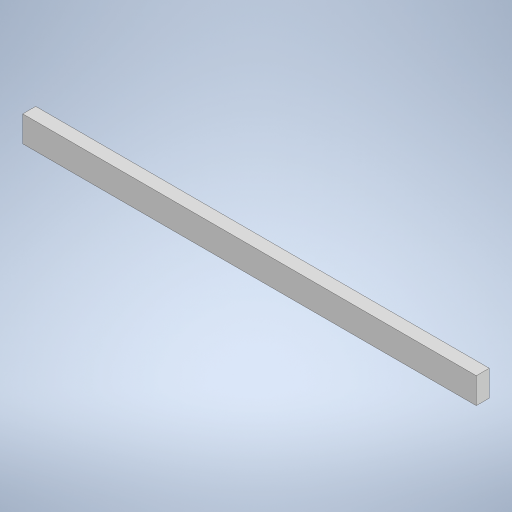
# Autodesk Inventor part: tail vertical rod
Saved by Autodesk Inventor 2024 (Build 280153000, 153)
## iProperties
Created: 2023-07-07
Part Number: tail vertical rod
Material: Generic
Document SubType Name: Modeling
Designer: USER
Density: 1 g/cm^3
Appearance: Default
Author: USER
Autodesk Inventor part; units mm, degrees
ref_plane "YZ Plane" through (0, 0, 0) normal (1, 0, 0) x (0, 1, 0)
ref_plane "XZ Plane" through (0, 0, 0) normal (0, 1, 0) x (-1, 0, 0)
ref_plane "XY Plane" through (0, 0, 0) normal (0, 0, 1) x (1, 0, 0)
sketch "Sketch1" plane through (0, 0, 0) normal (0, 0, 1) x (1, 0, 0)
  line L0 (150, 5) -> (-150, 5)
  line L1 (-150, 5) -> (-150, -5)
  line L2 (-150, -5) -> (150, -5)
  line L3 (150, -5) -> (150, 5)
  point P0 (0, 0)
  constraints: 8 end point, 2 parallel, 1 horizontal, 1 perpendicular
extrude "Extrusion1" add sketch "Sketch1" along normal blind 5
sketch "Sketch2" plane through (150, -5, 0) normal (1, 0, 0) x (0, 0, -1)
  line L0 (0, 0) -> (0, 10) projected
  line L1 (0, 10) -> (-5, 10) projected
  line L2 (-5, 0) -> (-5, 10) projected
  line L3 (0, 0) -> (-5, 0) projected
  point P0 (0, 5)
extrude "Extrusion2" cut sketch "Sketch2" against normal blind 150
sketch "Sketch3" plane through (0, -5, 0) normal (1, 0, 0) x (0, 0, -1)
  line L0 (0, 10) -> (0, 0) projected
  line L1 (-5, 10) -> (0, 10) projected
  line L2 (-5, 0) -> (-5, 10) projected
  line L3 (0, 0) -> (-5, 0) projected
  point P0 (0, 5)
extrude "Extrusion3" add sketch "Sketch3" along normal blind 50
sketch "Sketch4" plane through (50, -5, 0) normal (1, 0, 0) x (0, 0, -1)
  line L0 (-5, 10) -> (-5, 0) projected
  line L1 (-5, 0) -> (0, 0) projected
  line L2 (0, 0) -> (0, 10) projected
  line L3 (0, 10) -> (-5, 10) projected
  point P0 (0, 5)
extrude "Extrusion4" cut sketch "Sketch4" against normal blind 25
body "Solid1"
